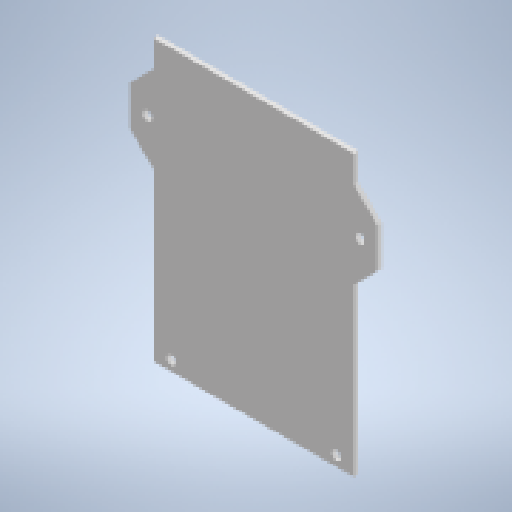
# Autodesk Inventor part: Cover
Saved by Autodesk Inventor 2024.2 (Build 282272000, 272)
## iProperties
Created: 2024-06-02
Part Number: Cover
Material: PBT Plastic
Document SubType Name: Modeling
Designer: simon
Density: 1.31 g/cm^3
Appearance: Cadet Blue
Author: simon
Autodesk Inventor part; units mm, degrees
ref_plane "YZ Plane" through (0, 0, 0) normal (1, 0, 0) x (0, 1, 0)
ref_plane "XZ Plane" through (0, 0, 0) normal (0, 1, 0) x (-1, 0, 0)
ref_plane "XY Plane" through (0, 0, 0) normal (0, 0, 1) x (1, 0, 0)
sketch "Sketch3" plane through (0, 0, 0) normal (0, 0, 1) x (1, 0, 0)
  line L0 (-10, 81) -> (0, 71) projected
  line L1 (-10, 96) -> (-10, 81) projected
  line L2 (0, 106) -> (-10, 96) projected
  line L3 (0, 116) -> (0, 106) projected
  line L4 (80, 116) -> (0, 116) projected
  line L5 (80, 106) -> (80, 116) projected
  line L6 (90, 96) -> (80, 106) projected
  line L7 (90, 81) -> (90, 96) projected
  line L8 (80, 71) -> (90, 81) projected
  line L9 (80, -0.1962) -> (80, 71) projected
  circle A0 centre (85, 88.5) radius 1.95 projected
  circle A1 centre (75, 4) radius 1.95 projected
  circle A2 centre (5, 4) radius 1.95 projected
  circle A3 centre (-5, 88.5) radius 1.95 projected
  line L10 (80, -0.1962) -> (80, 71)
  line L11 (80, 71) -> (90, 81)
  line L12 (90, 81) -> (90, 96)
  line L13 (90, 96) -> (80, 106)
  line L14 (80, 106) -> (80, 116)
  line L15 (80, 116) -> (0, 116)
  line L16 (0, 116) -> (0, 106)
  line L17 (0, 106) -> (-10, 96)
  line L18 (-10, 96) -> (-10, 81)
  line L19 (-10, 81) -> (0, 71)
  line L20 (80, -0.1962) -> (0, -0.1962)
  line L21 (0, 71) -> (0, -0.1962) projected
  line L22 (0, -0.1962) -> (0, 71)
  circle A4 centre (5, 4) radius 1.65
  circle A5 centre (-5, 88.5) radius 1.65
  circle A6 centre (85, 88.5) radius 1.65
  circle A7 centre (75, 4) radius 1.65
  line L23 (0, -0.1962) -> (-2.3, -0.1962)
  line L24 (-2.3, -0.1962) -> (-2.3, 70.0473)
  line L25 (-2.3, 70.0473) -> (-12.3, 80.0473)
  line L26 (-12.3, 80.0473) -> (-12.3, 96.9527)
  line L27 (-12.3, 96.9527) -> (-2.3, 106.9527)
  line L28 (-2.3, 106.9527) -> (-2.3, 118.3)
  line L29 (-2.3, 118.3) -> (82.3, 118.3)
  line L30 (82.3, 118.3) -> (82.3, 106.9527)
  line L31 (82.3, 106.9527) -> (92.3, 96.9527)
  line L32 (92.3, 96.9527) -> (92.3, 80.0473)
  line L33 (92.3, 80.0473) -> (82.3, 70.0473)
  line L34 (82.3, 70.0473) -> (82.3, -0.1962)
  line L35 (82.3, -0.1962) -> (80, -0.1962)
  point P0 (0, 0)
  dimension "d10" = 3.3
  dimension "d11" = 3.3
  dimension "d12" = 3.3
  dimension "d13" = 3.3
  dimension "d14" = 2.3
  dimension "d15" = 2.3
  dimension "d16" = 2.3
  dimension "d17" = 2.3
  dimension "d18" = 2.3
  dimension "d19" = 2.3
  dimension "d20" = 2.3
  dimension "d21" = 2.3
  dimension "d22" = 2.3
  dimension "d23" = 2.3
  dimension "d24" = 2.3
  constraints: 50 end point, 12 parallel, 10 perpendicular, 7 collinear, 4 centre point, 4 coincident, 1 horizontal, 1 point on line, 1 vertical
  measures "d10" diameter of A4
  measures "d11" diameter of A5
  measures "d12" diameter of A6
  measures "d13" diameter of A7
  measures "d14" distance of L20.end L23.end
  measures "d15" distance between parallel lines of L25 L0
  measures "d16" distance between parallel lines of L26 L1
  measures "d17" distance between parallel lines of L27 L2
  measures "d18" distance between parallel lines of L28 L3
  measures "d19" distance between parallel lines of L29 L4
  measures "d20" distance between parallel lines of L30 L5
  measures "d21" distance between parallel lines of L6 L31
  measures "d22" distance between parallel lines of L7 L32
  measures "d23" distance between parallel lines of L33 L11
  measures "d24" distance between parallel lines of L9 L34
extrude "Extrusion2" add sketch "Sketch3" along normal blind 2 contours L1 L2 L3 L4 L5 L6 L7 L8 L9 L20 L21 L0 | L0 L21 L23 L24 L25 L26 L27 L28 L29 L30 L31 L32 L33 L34 L35 L9 L8 L7 L6 L5 L4 L3 L2 L1
body "Solid2"
